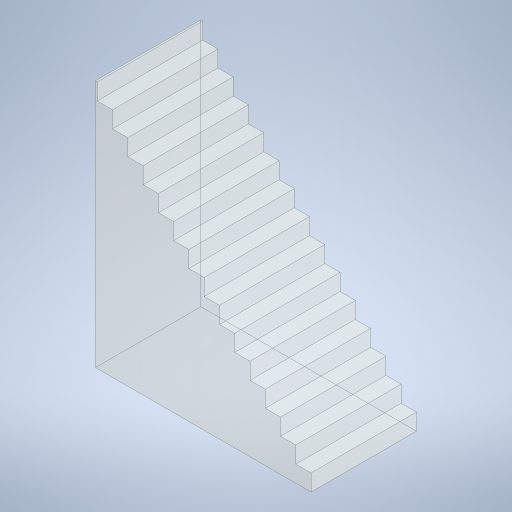
# Autodesk Inventor part: Stairs_Between_Finished_Basement_And_First_Floor
Saved by Autodesk Inventor 2024 (Build 280153000, 153)
## iProperties
Created: 2023-05-16
Part Number: Stairs_Between_Finished_Basement_And_First_Floor
Material: Wood (Southern Pine)
Document SubType Name: Modeling
Designer: Tom
Density: 0.420735 g/cm^3
Appearance: Clear
Mass: 2.17052e+07 g
Surface Area: 147038 cm^2
Volume: 2.765e+06 cm^3
Author: Tom
Autodesk Inventor part; units mm, degrees
ref_plane "YZ Plane" through (0, 0, 0) normal (1, 0, 0) x (0, 1, 0)
ref_plane "XZ Plane" through (0, 0, 0) normal (0, 1, 0) x (-1, 0, 0)
ref_plane "XY Plane" through (0, 0, 0) normal (0, 0, 1) x (1, 0, 0)
sketch "Sketch1" plane through (0, 0, 0) normal (0, 0, 1) x (1, 0, 0)
  line L0 (-162.8321, 176.53) -> (-162.8321, 353.06)
  line L1 (-162.8321, 353.06) -> (-325.6643, 353.06)
  line L2 (-325.6643, 353.06) -> (-325.6643, 529.59)
  line L3 (-325.6643, 529.59) -> (-488.4964, 529.59)
  line L4 (-488.4964, 529.59) -> (-488.4964, 706.12)
  line L5 (-488.4964, 706.12) -> (-651.3286, 706.12)
  line L6 (-651.3286, 706.12) -> (-651.3286, 882.65)
  line L7 (-651.3286, 882.65) -> (-814.1607, 882.65)
  line L8 (-814.1607, 882.65) -> (-814.1607, 1059.18)
  line L9 (-814.1607, 1059.18) -> (-976.9929, 1059.18)
  line L10 (-976.9929, 1059.18) -> (-976.9929, 1235.71)
  line L11 (-976.9929, 1235.71) -> (-1139.825, 1235.71)
  line L12 (-1139.825, 1235.71) -> (-1139.825, 1412.24)
  line L13 (-1139.825, 1412.24) -> (-1302.6571, 1412.24)
  line L14 (-1302.6571, 1412.24) -> (-1302.6571, 1588.77)
  line L15 (-1302.6571, 1588.77) -> (-1465.4893, 1588.77)
  line L16 (-1465.4893, 1588.77) -> (-1465.4893, 1765.3)
  line L17 (-1465.4893, 1765.3) -> (-1628.3214, 1765.3)
  line L18 (-1628.3214, 1765.3) -> (-1628.3214, 1941.83)
  line L19 (-1628.3214, 1941.83) -> (-1791.1536, 1941.83)
  line L20 (-1791.1536, 1941.83) -> (-1791.1536, 2118.36)
  line L21 (-1791.1536, 2118.36) -> (-1953.9857, 2118.36)
  line L22 (-1953.9857, 2118.36) -> (-1953.9857, 2294.89)
  line L23 (-1953.9857, 2294.89) -> (-2116.8179, 2294.89)
  line L24 (-162.8321, 176.53) -> (0, 176.53)
  line L25 (0, 176.53) -> (0, 0)
  line L26 (0, 0) -> (-2298.7, 0)
  line L27 (-2116.8179, 2294.89) -> (-2116.8179, 2471.42)
  line L28 (-2116.8179, 2471.42) -> (-2279.65, 2471.42)
  line L29 (-2279.65, 2471.42) -> (-2279.65, 2647.95)
  line L30 (-2279.65, 2647.95) -> (-2298.7, 2647.95)
  line L31 (-2298.7, 2647.95) -> (-2298.7, 0)
  point P0 (-2762.8302, 625.5305)
  dimension "d21" = 2647.95
  dimension "d22" = 2298.7
  dimension "d23" = 19.05
  constraints: 64 end point, 27 parallel, 26 perpendicular, 3 horizontal, 3 vertical, 1 coincident
  measures "d21" distance of L30.end L26.end
  measures "d22" distance of L25.end L26.end
  measures "d23" distance of L29.end L30.end
extrude "Extrusion1" add sketch "Sketch1" along normal blind 1123.95
body "Solid1"
